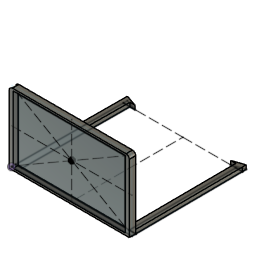
LightSwitchShelf (Autodesk Fusion 360 design; units mm, degrees)
Autodesk Fusion 360 part; units mm, degrees
sketch "Sketch1" plane through (0, 0, 0) normal (0, 0, 1) x (1, 0, 0) in component "LightSwitchShelf"
  line L0 (0, 0) -> (93.15, 0)
  line L1 (93.15, 0) -> (93.15, 3)
  line L2 (93.15, 3) -> (0, 3)
  line L3 (0, 3) -> (0, 0)
  line L4 (0, 3) -> (5, 3)
  line L5 (93.15, 3) -> (88.15, 3)
  line L6 (46.575, 3) -> (46.575, 86.15) construction
  line L7 (0.5, 86.15) -> (46.575, 86.15) construction
  line L8 (46.575, 86.15) -> (92.65, 86.15) construction
  line L9 (0.5, 86.15) -> (5.5, 86.15)
  line L10 (92.65, 86.15) -> (87.65, 86.15)
  line L11 (0.5, 86.15) -> (0, 3)
  line L12 (5, 3) -> (5.5, 86.15)
  line L13 (87.65, 86.15) -> (88.15, 3)
  line L14 (93.15, 3) -> (92.65, 86.15)
  line L15 (0.5, 86.15) -> (9.4998, 86.0959)
  line L16 (0.5, 86.15) -> (0.518, 89.1499)
  line L17 (0.518, 89.1499) -> (9.4998, 86.0959)
  line L18 (92.65, 86.15) -> (83.6502, 86.0959)
  line L19 (92.65, 86.15) -> (92.65, 89.15)
  line L20 (92.65, 89.15) -> (83.6502, 86.0959)
  dimension "d2" = 3
  dimension "d8" = 5
  dimension "d10" = 83.15
  dimension "d11" = 46.075
  dimension "d14" = 9
  dimension "d15" = 3
  dimension "d17" = 3
  dimension "d18" = 90
  dimension "d19" = 90
  dimension "d29" = 83.15
  dimension "d30" = 82.15
  constraint horizontal L0
  constraint vertical L1
  constraint horizontal L2
  constraint vertical L3
  constraint coincident L0.start L3.end
  constraint perpendicular L3 L4
  constraint perpendicular L1 L5
  constraint midpoint L2 L6.start
  constraint perpendicular L2 L6
  constraint perpendicular L6 L7
  constraint perpendicular L6 L8
  constraint equal L7 L8
  constraint parallel L7 L9
  constraint parallel L8 L10
  constraint equal L4 L5
  constraint equal L4 L9
  constraint equal L5 L10
  constraint perpendicular L12 L15
  constraint perpendicular L15 L16
  constraint perpendicular L13 L18
  constraint perpendicular L10 L19
  constraint equal L15 L18
  measures "d2" distance of L0.start L2.end
  measures "d8" distance of L2.end L4.end
  measures "d10" distance of L6.start L6.end
  measures "d11" distance of L6.end L7.start
  measures "d14" distance of L7.start L15.end
  measures "d15" distance of L7.start L16.end
  measures "d17" distance of L8.end L19.end
  measures "d18" angle of L12 L15
  measures "d19" angle of L13 L18
  measures "d29" distance of L4.end L5.end
  measures "d30" distance of L9.end L10.end
extrude "Extrude1" add sketch "Sketch1" along normal blind 3 makes body 1 in component "LightSwitchShelf"
extrude "Extrude2" add sketch "Sketch1" along normal blind 55 separate body contours L0 L1 L2 L3 L4 L5 makes body 2 in component "LightSwitchShelf"
sketch "Sketch2" plane through (0, 0, 0) normal (0, -1, 0) x (1, 0, 0) in component "LightSwitchShelf"
  line L0 (0, 0) -> (93.15, 0)
  line L1 (93.15, 0) -> (93.15, 55)
  line L2 (93.15, 55) -> (0, 55)
  line L3 (0, 55) -> (0, 0)
  line L4 (46.575, 55) -> (46.575, 0) construction
  line L5 (0, 27.5) -> (93.15, 27.5) construction
  line L6 (88.075, 3.5) -> (5.075, 3.5)
  line L7 (5.075, 3.5) -> (5.075, 51.5)
  line L8 (5.075, 51.5) -> (88.075, 51.5)
  line L9 (88.075, 51.5) -> (88.075, 3.5)
  line L10 (88.075, 3.5) -> (5.075, 51.5) construction
  line L11 (5.075, 3.5) -> (88.075, 51.5) construction
  point P0 (46.575, 27.5)
  dimension "d24" = 48
  dimension "d25" = 83
  constraint midpoint L2 L4.start
  constraint midpoint L0 L4.end
  constraint midpoint L3 L5.start
  constraint midpoint L1 L5.end
  constraint horizontal L6
  constraint perpendicular L6 L7
  constraint parallel L6 L8
  constraint parallel L7 L9
  constraint coincident L10 P0
  constraint coincident L11 P0
  constraint midpoint L5 P0
  measures "d24" distance of L6.end L7.end
  measures "d25" distance of L7 L9
extrude "Extrude3" add sketch "Sketch2" along normal blind 2 bodies 1 2 in component "LightSwitchShelf"
chamfer "Chamfer1" distance 2 angle 45 4 edges at (5.075, -2, 27.5) (46.575, -2, 51.5) (88.075, -2, 27.5) (46.575, -2, 3.5) on bodies 1 in component "LightSwitchShelf"
fillet "Fillet1" radius 2.5 2 edges at (0, 0.5, 55) (93.15, 0.5, 55) on bodies 1 in component "LightSwitchShelf"
component "LightSwitchShelf" placed x (1, 0, 0) y (0, 1, 0) z (0, 0, 1) at (0, 0, 0)
equation "d11 = ( 83.15 / 2 ) * 1 mm + 4.5 mm"
